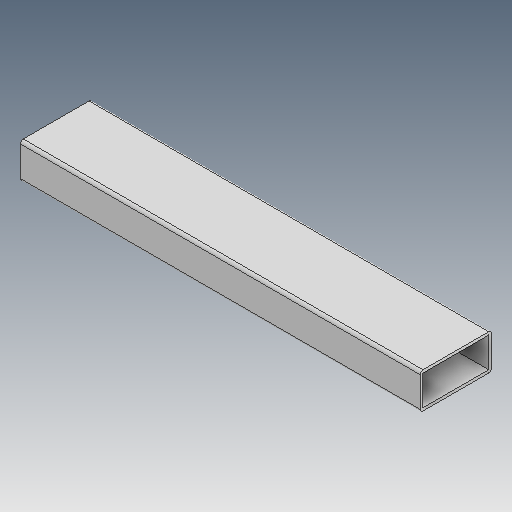
# Autodesk Inventor part: MC03-1
Saved by Autodesk Inventor 2020 (Build 240168000, 168)
## iProperties
Created: 2020-02-24
Part Number: MC03-1
Material: Generic
Document SubType Name: Modeling
Designer: Juan Carlos Botero
Density: 1 g/cm^3
Appearance: Default
Author: Juan Carlos Botero
Title: PERFIL REFUERZO BANDA
Autodesk Inventor part; units mm, degrees
ref_plane "YZ Plane" through (0, 0, 0) normal (1, 0, 0) x (0, 1, 0)
ref_plane "XZ Plane" through (0, 0, 0) normal (0, 1, 0) x (-1, 0, 0)
ref_plane "XY Plane" through (0, 0, 0) normal (0, 0, 1) x (1, 0, 0)
sketch "Sketch1" plane through (0, 0, 0) normal (1, 0, 0) x (0, 1, 0)
  line L0 (25, -50) -> (-25, -50)
  line L1 (-25, -50) -> (-25, 50)
  line L2 (-25, 50) -> (25, 50)
  line L3 (25, 50) -> (25, -50)
  line L4 (25, -50) -> (-25, 50) construction
  line L5 (-25, -50) -> (25, 50) construction
  point P0 (0, 0)
  dimension "d0" = 50
  dimension "d1" = 100
  constraints: 12 end point, 2 midpoint, 2 parallel, 1 horizontal, 1 perpendicular
  measures "d0" distance of L1.end L2.end
  measures "d1" distance of L0.end L1.end
extrude "Extrusion1" add sketch "Sketch1" along normal mid plane 559
fillet "Fillet1" radius 4 4 edges at (0, 25, 50) (0, -25, 50) (0, -25, -50) (0, 25, -50)
shell "Shell1" thickness 4 removed faces 2 at (-279.5, -8.3333, -15.3333) at (279.5, -8.3333, -15.3333)
body "Solid1"
